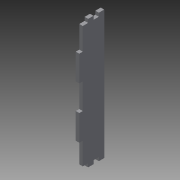
# Autodesk Inventor part: cajon front
Saved by Autodesk Inventor 2015 (Build 190159000, 159)
## iProperties
Created: 2016-01-26
Part Number: cajon front
Material: Generic
Document SubType Name: Modeling
Designer: iberopuebla
Density: 1 g/cm^3
Appearance: Default
Author: iberopuebla
Autodesk Inventor part; units mm, degrees
ref_plane "YZ Plane" through (0, 0, 0) normal (1, 0, 0) x (0, 1, 0)
ref_plane "XZ Plane" through (0, 0, 0) normal (0, 1, 0) x (-1, 0, 0)
ref_plane "XY Plane" through (0, 0, 0) normal (0, 0, 1) x (1, 0, 0)
sketch "Sketch1" plane through (0, 0, 0) normal (1, 0, 0) x (0, 1, 0)
  line L0 (27.5, 0) -> (55, 0)
  line L1 (110, 0) -> (110, -660)
  line L2 (55, -660) -> (27.5, -660)
  line L3 (0, -132) -> (-18, -132)
  line L4 (0, -264) -> (-18, -264)
  line L5 (0, -396) -> (-18, -396)
  line L6 (0, -528) -> (-18, -528)
  line L7 (-18, -132) -> (-18, -264)
  line L8 (-18, -396) -> (-18, -528)
  line L9 (0, -642) -> (0, -528)
  line L10 (0, -396) -> (0, -264)
  line L11 (0, -132) -> (0, -18)
  line L12 (55, -18) -> (55, 0)
  line L13 (27.5, -18) -> (27.5, 0)
  line L14 (0, -18) -> (27.5, -18)
  line L15 (55, -18) -> (82.5, -18)
  line L16 (55, -642) -> (55, -660)
  line L17 (27.5, -642) -> (27.5, -660)
  line L18 (0, -642) -> (27.5, -642)
  line L19 (55, -642) -> (82.5, -642)
  line L20 (82.5, -18) -> (82.5, 0)
  line L21 (82.5, 0) -> (110, 0)
  line L22 (82.5, -642) -> (82.5, -660)
  line L23 (82.5, -660) -> (110, -660)
  point P0 (0, 0)
  dimension "d3" = 132
  dimension "d4" = 132
  dimension "d5" = 132
  dimension "d6" = 132
  dimension "d8" = 18
  dimension "d9" = 18
  dimension "d10" = 18
  dimension "d17" = 660
  dimension "d22" = 18
  dimension "d35" = 18
  dimension "d36" = 18
  dimension "d37" = 18
  dimension "d38" = 18
  dimension "d39" = 18
  dimension "d41" = 18
  dimension "d46" = 27.5
  dimension "d47" = 27.5
  dimension "d48" = 27.5
  dimension "d49" = 27.5
  dimension "d50" = 27.5
  dimension "d51" = 27.5
  dimension "d52" = 27.5
  dimension "d53" = 27.5
  dimension "d54" = 110
  constraints: 48 end point, 19 perpendicular, 4 parallel, 4 vertical, 1 horizontal
  measures "d3" distance from line of point (0, 0) L3
  measures "d4" distance between parallel lines of L4 L3
  measures "d5" distance between parallel lines of L5 L4
  measures "d6" distance between parallel lines of L6 L5
  measures "d8" horizontal distance of L9.start L6.end
  measures "d9" distance of L5.start L5.end
  measures "d10" distance of L4.start L4.end
  measures "d17" distance between parallel lines of L2 L0
  measures "d22" distance of L13.start L0.start
  measures "d35" distance of L15.end L20.end
  measures "d36" distance of L12.start L0.end
  measures "d37" distance of L19.end L22.end
  measures "d38" distance of L16.start L2.start
  measures "d39" distance of L17.start L2.end
  measures "d41" distance from line of point (0, 0) L14
  measures "d46" distance of L11.end L13.start
  measures "d47" distance of L0.start L0.end
  measures "d48" distance of L12.start L15.end
  measures "d49" distance of L20.end L1.start
  measures "d50" distance of L9.start L17.start
  measures "d51" distance of L2.start L2.end
  measures "d52" distance of L16.start L19.end
  measures "d53" distance of L22.end L1.end
  measures "d54" distance from line of L1 point (0, 0)
extrude "Extrusion2" add sketch "Sketch1" along normal blind 18
body "Solid2"
